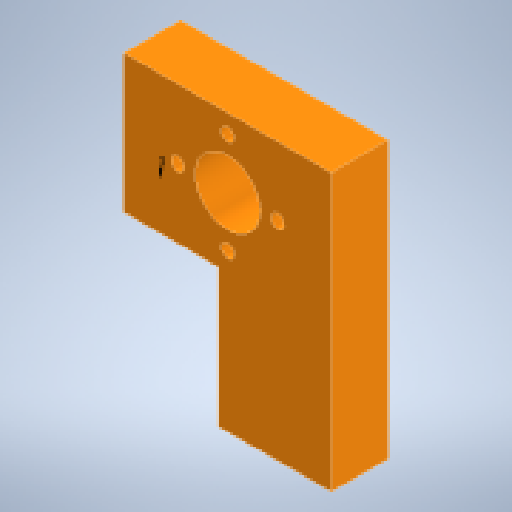
# Autodesk Inventor part: batente_microswitch_001
Saved by Autodesk Inventor 2026 (Build 300175000, 175)
## iProperties
Created: 2025-11-26
Part Number: batente_microswitch_001
Material: ABS Plastic
Document SubType Name: Modeling
Designer: Carlos Dias
Density: 1.06 g/cm^3
Appearance: Orange
Author: Carlos Dias
Autodesk Inventor part; units mm, degrees
ref_plane "YZ Plane" through (0, 0, 0) normal (1, 0, 0) x (0, 1, 0)
ref_plane "XZ Plane" through (0, 0, 0) normal (0, 1, 0) x (-1, 0, 0)
ref_plane "XY Plane" through (0, 0, 0) normal (0, 0, 1) x (1, 0, 0)
sketch "Sketch1" plane through (0, 0, 0) normal (0, 0, 1) x (1, 0, 0)
  line L0 (-16.5, 11) -> (16.5, 11)
  line L1 (16.5, 11) -> (16.5, -11)
  line L2 (16.5, -11) -> (-16.5, -11) construction
  line L3 (-16.5, -11) -> (-16.5, 11)
  line L4 (-16.5, 11) -> (16.5, -11) construction
  line L5 (16.5, 11) -> (-16.5, -11) construction
  line L6 (-16.5, -11) -> (-1.5, -11)
  line L7 (-1.5, -11) -> (-1.5, -33)
  line L8 (-1.5, -33) -> (16.5, -33)
  line L9 (16.5, -33) -> (16.5, -11)
  circle A0 centre (0, 0) radius 5.15
  circle A1 centre (0, 8) radius 1.05
  circle A2 centre (-8, 0) radius 1.05
  circle A3 centre (0, -8) radius 1.05
  circle A4 centre (8, 0) radius 1.05
  dimension "d0" = 33
  dimension "d1" = 22
  dimension "d2" = 15
  dimension "d3" = 44
  dimension "d4" = 10.3
  dimension "d5" = 8
  dimension "d8" = 360
  dimension "d10" = 2.1
  constraints: 20 end point, 5 centre point, 3 horizontal, 2 coincident, 2 midpoint, 2 parallel, 2 perpendicular, 1 vertical, 1 vertical alignment, 9 other
  measures "d0" distance of L0.start L0.end
  measures "d1" distance of L2.end L0.start
  measures "d2" distance of L2.end L6.end
  measures "d3" distance between parallel lines of L8 L0
  measures "d4" diameter of A0
  measures "d5" distance of point (0, 0) A1.centre
  measures "d10" diameter of A1
extrude "Extrusion1" add sketch "Sketch1" along normal blind 9
sketch "Sketch2" plane through (-16.5, -11, 0) normal (-1, 0, 0) x (0, 0, 1)
  circle A0 centre (4.5, 4) radius 1.5
  line L0 (0, 0) -> (9, 0) construction
  line L1 (9, 22) -> (9, 0) projected
  line L2 (0, 11) -> (9, 11) construction
  line L3 (0, 22) -> (0, 0) projected
  circle A1 centre (4.5, 18) radius 1.5
  point P0 (0, 11)
  point P1 (4.5, 0)
  dimension "d13" = 3
  dimension "d14" = 4
  constraints: 4 end point, 3 midpoint, 2 centre point, 2 horizontal, 1 coincident, 1 point on line, 1 symmetric about line, 1 vertical alignment, 1 other
  measures "d13" diameter of A0
  measures "d14" distance from line of A0.centre L0
extrude "Extrusion2" cut sketch "Sketch2" against normal blind 5
body "Solid1"
